Autodesk Fusion 360 part; units mm, degrees
(part 5 of 6)
  arc A300 (17.675, -158.5) -> (14.5, -161.675) centre (17.675, -161.675) ccw
  line L301 (17.675, -158.5) -> (30.325, -158.5)
  arc A301 (33.5, -161.675) -> (30.325, -158.5) centre (30.325, -161.675) ccw
  line L302 (33.5, -161.675) -> (33.5, -174.325)
  arc A302 (30.325, -177.5) -> (33.5, -174.325) centre (30.325, -174.325) ccw
  line L303 (30.325, -177.5) -> (17.675, -177.5)
  arc A303 (14.5, -174.325) -> (17.675, -177.5) centre (17.675, -174.325) ccw
  line L304 (-105.5, -126.325) -> (-105.5, -113.675)
  arc A304 (-102.325, -110.5) -> (-105.5, -113.675) centre (-102.325, -113.675) ccw
  line L305 (-102.325, -110.5) -> (-89.675, -110.5)
  arc A305 (-86.5, -113.675) -> (-89.675, -110.5) centre (-89.675, -113.675) ccw
  line L306 (-86.5, -113.675) -> (-86.5, -126.325)
  arc A306 (-89.675, -129.5) -> (-86.5, -126.325) centre (-89.675, -126.325) ccw
  line L307 (-89.675, -129.5) -> (-102.325, -129.5)
  arc A307 (-105.5, -126.325) -> (-102.325, -129.5) centre (-102.325, -126.325) ccw
  line L308 (-81.5, -6.325) -> (-81.5, 6.325)
  arc A308 (-78.325, 9.5) -> (-81.5, 6.325) centre (-78.325, 6.325) ccw
  line L309 (-78.325, 9.5) -> (-65.675, 9.5)
  arc A309 (-62.5, 6.325) -> (-65.675, 9.5) centre (-65.675, 6.325) ccw
  line L310 (-62.5, 6.325) -> (-62.5, -6.325)
  arc A310 (-65.675, -9.5) -> (-62.5, -6.325) centre (-65.675, -6.325) ccw
  line L311 (-65.675, -9.5) -> (-78.325, -9.5)
  arc A311 (-81.5, -6.325) -> (-78.325, -9.5) centre (-78.325, -6.325) ccw
  line L312 (-33.5, -102.325) -> (-33.5, -89.675)
  arc A312 (-30.325, -86.5) -> (-33.5, -89.675) centre (-30.325, -89.675) ccw
  line L313 (-30.325, -86.5) -> (-17.675, -86.5)
  arc A313 (-14.5, -89.675) -> (-17.675, -86.5) centre (-17.675, -89.675) ccw
  line L314 (-14.5, -89.675) -> (-14.5, -102.325)
  arc A314 (-17.675, -105.5) -> (-14.5, -102.325) centre (-17.675, -102.325) ccw
  line L315 (-17.675, -105.5) -> (-30.325, -105.5)
  arc A315 (-33.5, -102.325) -> (-30.325, -105.5) centre (-30.325, -102.325) ccw
  line L316 (-81.5, -126.325) -> (-81.5, -113.675)
  arc A316 (-78.325, -110.5) -> (-81.5, -113.675) centre (-78.325, -113.675) ccw
  line L317 (-78.325, -110.5) -> (-65.675, -110.5)
  arc A317 (-62.5, -113.675) -> (-65.675, -110.5) centre (-65.675, -113.675) ccw
  line L318 (-62.5, -113.675) -> (-62.5, -126.325)
  arc A318 (-65.675, -129.5) -> (-62.5, -126.325) centre (-65.675, -126.325) ccw
  line L319 (-65.675, -129.5) -> (-78.325, -129.5)
  arc A319 (-81.5, -126.325) -> (-78.325, -129.5) centre (-78.325, -126.325) ccw
  line L320 (38.5, 161.675) -> (38.5, 174.325)
  arc A320 (41.675, 177.5) -> (38.5, 174.325) centre (41.675, 174.325) ccw
  line L321 (41.675, 177.5) -> (54.325, 177.5)
  arc A321 (57.5, 174.325) -> (54.325, 177.5) centre (54.325, 174.325) ccw
  line L322 (57.5, 174.325) -> (57.5, 161.675)
  arc A322 (54.325, 158.5) -> (57.5, 161.675) centre (54.325, 161.675) ccw
  line L323 (54.325, 158.5) -> (41.675, 158.5)
  arc A323 (38.5, 161.675) -> (41.675, 158.5) centre (41.675, 161.675) ccw
  line L324 (38.5, 137.675) -> (38.5, 150.325)
  arc A324 (41.675, 153.5) -> (38.5, 150.325) centre (41.675, 150.325) ccw
  line L325 (41.675, 153.5) -> (54.325, 153.5)
  arc A325 (57.5, 150.325) -> (54.325, 153.5) centre (54.325, 150.325) ccw
  line L326 (57.5, 150.325) -> (57.5, 137.675)
  arc A326 (54.325, 134.5) -> (57.5, 137.675) centre (54.325, 137.675) ccw
  line L327 (54.325, 134.5) -> (41.675, 134.5)
  arc A327 (38.5, 137.675) -> (41.675, 134.5) centre (41.675, 137.675) ccw
  line L328 (38.5, 113.675) -> (38.5, 126.325)
  arc A328 (41.675, 129.5) -> (38.5, 126.325) centre (41.675, 126.325) ccw
  line L329 (41.675, 129.5) -> (54.325, 129.5)
  arc A329 (57.5, 126.325) -> (54.325, 129.5) centre (54.325, 126.325) ccw
  line L330 (57.5, 126.325) -> (57.5, 113.675)
  arc A330 (54.325, 110.5) -> (57.5, 113.675) centre (54.325, 113.675) ccw
  line L331 (54.325, 110.5) -> (41.675, 110.5)
  arc A331 (38.5, 113.675) -> (41.675, 110.5) centre (41.675, 113.675) ccw
  line L332 (38.5, 89.675) -> (38.5, 102.325)
  arc A332 (41.675, 105.5) -> (38.5, 102.325) centre (41.675, 102.325) ccw
  line L333 (41.675, 105.5) -> (54.325, 105.5)
  arc A333 (57.5, 102.325) -> (54.325, 105.5) centre (54.325, 102.325) ccw
  line L334 (57.5, 102.325) -> (57.5, 89.675)
  arc A334 (54.325, 86.5) -> (57.5, 89.675) centre (54.325, 89.675) ccw
  line L335 (54.325, 86.5) -> (41.675, 86.5)
  arc A335 (38.5, 89.675) -> (41.675, 86.5) centre (41.675, 89.675) ccw
  line L336 (134.5, 161.675) -> (134.5, 174.325)
  arc A336 (137.675, 177.5) -> (134.5, 174.325) centre (137.675, 174.325) ccw
  line L337 (137.675, 177.5) -> (150.325, 177.5)
  arc A337 (153.5, 174.325) -> (150.325, 177.5) centre (150.325, 174.325) ccw
  line L338 (153.5, 174.325) -> (153.5, 161.675)
  arc A338 (150.325, 158.5) -> (153.5, 161.675) centre (150.325, 161.675) ccw
  line L339 (150.325, 158.5) -> (137.675, 158.5)
  arc A339 (134.5, 161.675) -> (137.675, 158.5) centre (137.675, 161.675) ccw
  line L340 (62.5, 41.675) -> (62.5, 54.325)
  arc A340 (65.675, 57.5) -> (62.5, 54.325) centre (65.675, 54.325) ccw
  line L341 (65.675, 57.5) -> (78.325, 57.5)
  arc A341 (81.5, 54.325) -> (78.325, 57.5) centre (78.325, 54.325) ccw
  line L342 (81.5, 54.325) -> (81.5, 41.675)
  arc A342 (78.325, 38.5) -> (81.5, 41.675) centre (78.325, 41.675) ccw
  line L343 (78.325, 38.5) -> (65.675, 38.5)
  arc A343 (62.5, 41.675) -> (65.675, 38.5) centre (65.675, 41.675) ccw
  line L344 (62.5, 17.675) -> (62.5, 30.325)
  arc A344 (65.675, 33.5) -> (62.5, 30.325) centre (65.675, 30.325) ccw
  line L345 (65.675, 33.5) -> (78.325, 33.5)
  arc A345 (81.5, 30.325) -> (78.325, 33.5) centre (78.325, 30.325) ccw
  line L346 (81.5, 30.325) -> (81.5, 17.675)
  arc A346 (78.325, 14.5) -> (81.5, 17.675) centre (78.325, 17.675) ccw
  line L347 (78.325, 14.5) -> (65.675, 14.5)
  arc A347 (62.5, 17.675) -> (65.675, 14.5) centre (65.675, 17.675) ccw
  line L348 (62.5, -6.325) -> (62.5, 6.325)
  arc A348 (65.675, 9.5) -> (62.5, 6.325) centre (65.675, 6.325) ccw
  line L349 (65.675, 9.5) -> (78.325, 9.5)
  arc A349 (81.5, 6.325) -> (78.325, 9.5) centre (78.325, 6.325) ccw
  line L350 (81.5, 6.325) -> (81.5, -6.325)
  arc A350 (78.325, -9.5) -> (81.5, -6.325) centre (78.325, -6.325) ccw
  line L351 (78.325, -9.5) -> (65.675, -9.5)
  arc A351 (62.5, -6.325) -> (65.675, -9.5) centre (65.675, -6.325) ccw
  line L352 (158.5, 161.675) -> (158.5, 174.325)
  arc A352 (161.675, 177.5) -> (158.5, 174.325) centre (161.675, 174.325) ccw
  line L353 (161.675, 177.5) -> (174.325, 177.5)
  arc A353 (177.5, 174.325) -> (174.325, 177.5) centre (174.325, 174.325) ccw
  line L354 (177.5, 174.325) -> (177.5, 161.675)
  arc A354 (174.325, 158.5) -> (177.5, 161.675) centre (174.325, 161.675) ccw
  line L355 (174.325, 158.5) -> (161.675, 158.5)
  arc A355 (158.5, 161.675) -> (161.675, 158.5) centre (161.675, 161.675) ccw
  line L356 (134.5, 137.675) -> (134.5, 150.325)
  arc A356 (137.675, 153.5) -> (134.5, 150.325) centre (137.675, 150.325) ccw
  line L357 (137.675, 153.5) -> (150.325, 153.5)
  arc A357 (153.5, 150.325) -> (150.325, 153.5) centre (150.325, 150.325) ccw
  line L358 (153.5, 150.325) -> (153.5, 137.675)
  arc A358 (150.325, 134.5) -> (153.5, 137.675) centre (150.325, 137.675) ccw
  line L359 (150.325, 134.5) -> (137.675, 134.5)
  arc A359 (134.5, 137.675) -> (137.675, 134.5) centre (137.675, 137.675) ccw
  line L360 (134.5, 113.675) -> (134.5, 126.325)
  arc A360 (137.675, 129.5) -> (134.5, 126.325) centre (137.675, 126.325) ccw
  line L361 (137.675, 129.5) -> (150.325, 129.5)
  arc A361 (153.5, 126.325) -> (150.325, 129.5) centre (150.325, 126.325) ccw
  line L362 (153.5, 126.325) -> (153.5, 113.675)
  arc A362 (150.325, 110.5) -> (153.5, 113.675) centre (150.325, 113.675) ccw
  line L363 (150.325, 110.5) -> (137.675, 110.5)
  arc A363 (134.5, 113.675) -> (137.675, 110.5) centre (137.675, 113.675) ccw
  line L364 (134.5, 89.675) -> (134.5, 102.325)
  arc A364 (137.675, 105.5) -> (134.5, 102.325) centre (137.675, 102.325) ccw
  line L365 (137.675, 105.5) -> (150.325, 105.5)
  arc A365 (153.5, 102.325) -> (150.325, 105.5) centre (150.325, 102.325) ccw
  line L366 (153.5, 102.325) -> (153.5, 89.675)
  arc A366 (150.325, 86.5) -> (153.5, 89.675) centre (150.325, 89.675) ccw
  line L367 (150.325, 86.5) -> (137.675, 86.5)
  arc A367 (134.5, 89.675) -> (137.675, 86.5) centre (137.675, 89.675) ccw
  line L368 (134.5, 65.675) -> (134.5, 78.325)
  arc A368 (137.675, 81.5) -> (134.5, 78.325) centre (137.675, 78.325) ccw
  line L369 (137.675, 81.5) -> (150.325, 81.5)
  arc A369 (153.5, 78.325) -> (150.325, 81.5) centre (150.325, 78.325) ccw
  line L370 (153.5, 78.325) -> (153.5, 65.675)
  arc A370 (150.325, 62.5) -> (153.5, 65.675) centre (150.325, 65.675) ccw
  line L371 (150.325, 62.5) -> (137.675, 62.5)
  arc A371 (134.5, 65.675) -> (137.675, 62.5) centre (137.675, 65.675) ccw
  line L372 (134.5, 41.675) -> (134.5, 54.325)
  arc A372 (137.675, 57.5) -> (134.5, 54.325) centre (137.675, 54.325) ccw
  line L373 (137.675, 57.5) -> (150.325, 57.5)
  arc A373 (153.5, 54.325) -> (150.325, 57.5) centre (150.325, 54.325) ccw
  line L374 (153.5, 54.325) -> (153.5, 41.675)
  arc A374 (150.325, 38.5) -> (153.5, 41.675) centre (150.325, 41.675) ccw
  line L375 (150.325, 38.5) -> (137.675, 38.5)
  arc A375 (134.5, 41.675) -> (137.675, 38.5) centre (137.675, 41.675) ccw
  line L376 (134.5, 17.675) -> (134.5, 30.325)
  arc A376 (137.675, 33.5) -> (134.5, 30.325) centre (137.675, 30.325) ccw
  line L377 (137.675, 33.5) -> (150.325, 33.5)
  arc A377 (153.5, 30.325) -> (150.325, 33.5) centre (150.325, 30.325) ccw
  line L378 (153.5, 30.325) -> (153.5, 17.675)
  arc A378 (150.325, 14.5) -> (153.5, 17.675) centre (150.325, 17.675) ccw
  line L379 (150.325, 14.5) -> (137.675, 14.5)
  arc A379 (134.5, 17.675) -> (137.675, 14.5) centre (137.675, 17.675) ccw
  line L380 (134.5, -6.325) -> (134.5, 6.325)
  arc A380 (137.675, 9.5) -> (134.5, 6.325) centre (137.675, 6.325) ccw
  line L381 (137.675, 9.5) -> (150.325, 9.5)
  arc A381 (153.5, 6.325) -> (150.325, 9.5) centre (150.325, 6.325) ccw
  line L382 (153.5, 6.325) -> (153.5, -6.325)
  arc A382 (150.325, -9.5) -> (153.5, -6.325) centre (150.325, -6.325) ccw
  line L383 (150.325, -9.5) -> (137.675, -9.5)
  arc A383 (134.5, -6.325) -> (137.675, -9.5) centre (137.675, -6.325) ccw
  line L384 (38.5, -30.325) -> (38.5, -17.675)
  arc A384 (41.675, -14.5) -> (38.5, -17.675) centre (41.675, -17.675) ccw
  line L385 (41.675, -14.5) -> (54.325, -14.5)
  arc A385 (57.5, -17.675) -> (54.325, -14.5) centre (54.325, -17.675) ccw
  line L386 (57.5, -17.675) -> (57.5, -30.325)
  arc A386 (54.325, -33.5) -> (57.5, -30.325) centre (54.325, -30.325) ccw
  line L387 (54.325, -33.5) -> (41.675, -33.5)
  arc A387 (38.5, -30.325) -> (41.675, -33.5) centre (41.675, -30.325) ccw
  line L388 (38.5, -54.325) -> (38.5, -41.675)
  arc A388 (41.675, -38.5) -> (38.5, -41.675) centre (41.675, -41.675) ccw
  line L389 (41.675, -38.5) -> (54.325, -38.5)
  arc A389 (57.5, -41.675) -> (54.325, -38.5) centre (54.325, -41.675) ccw
  line L390 (57.5, -41.675) -> (57.5, -54.325)
  arc A390 (54.325, -57.5) -> (57.5, -54.325) centre (54.325, -54.325) ccw
  line L391 (54.325, -57.5) -> (41.675, -57.5)
  arc A391 (38.5, -54.325) -> (41.675, -57.5) centre (41.675, -54.325) ccw
  line L392 (-9.5, -102.325) -> (-9.5, -89.675)
  arc A392 (-6.325, -86.5) -> (-9.5, -89.675) centre (-6.325, -89.675) ccw
  line L393 (-6.325, -86.5) -> (6.325, -86.5)
  arc A393 (9.5, -89.675) -> (6.325, -86.5) centre (6.325, -89.675) ccw
  line L394 (9.5, -89.675) -> (9.5, -102.325)
  arc A394 (6.325, -105.5) -> (9.5, -102.325) centre (6.325, -102.325) ccw
  line L395 (6.325, -105.5) -> (-6.325, -105.5)
  arc A395 (-9.5, -102.325) -> (-6.325, -105.5) centre (-6.325, -102.325) ccw
  line L396 (134.5, -78.325) -> (134.5, -65.675)
  arc A396 (137.675, -62.5) -> (134.5, -65.675) centre (137.675, -65.675) ccw
  line L397 (137.675, -62.5) -> (150.325, -62.5)
  arc A397 (153.5, -65.675) -> (150.325, -62.5) centre (150.325, -65.675) ccw
  line L398 (153.5, -65.675) -> (153.5, -78.325)
  arc A398 (150.325, -81.5) -> (153.5, -78.325) centre (150.325, -78.325) ccw
  line L399 (150.325, -81.5) -> (137.675, -81.5)
  arc A399 (134.5, -78.325) -> (137.675, -81.5) centre (137.675, -78.325) ccw
  line L400 (-33.5, 17.675) -> (-33.5, 30.325)
  arc A400 (-30.325, 33.5) -> (-33.5, 30.325) centre (-30.325, 30.325) ccw
  line L401 (-30.325, 33.5) -> (-17.675, 33.5)
  arc A401 (-14.5, 30.325) -> (-17.675, 33.5) centre (-17.675, 30.325) ccw
  line L402 (-14.5, 30.325) -> (-14.5, 17.675)
  arc A402 (-17.675, 14.5) -> (-14.5, 17.675) centre (-17.675, 17.675) ccw
  line L403 (-17.675, 14.5) -> (-30.325, 14.5)
  arc A403 (-33.5, 17.675) -> (-30.325, 14.5) centre (-30.325, 17.675) ccw
  line L404 (62.5, -78.325) -> (62.5, -65.675)
  arc A404 (65.675, -62.5) -> (62.5, -65.675) centre (65.675, -65.675) ccw
  line L405 (65.675, -62.5) -> (78.325, -62.5)
  arc A405 (81.5, -65.675) -> (78.325, -62.5) centre (78.325, -65.675) ccw
  line L406 (81.5, -65.675) -> (81.5, -78.325)
  arc A406 (78.325, -81.5) -> (81.5, -78.325) centre (78.325, -78.325) ccw
  line L407 (78.325, -81.5) -> (65.675, -81.5)
  arc A407 (62.5, -78.325) -> (65.675, -81.5) centre (65.675, -78.325) ccw
  line L408 (-153.5, 17.675) -> (-153.5, 30.325)
  arc A408 (-150.325, 33.5) -> (-153.5, 30.325) centre (-150.325, 30.325) ccw
  line L409 (-150.325, 33.5) -> (-137.675, 33.5)
  arc A409 (-134.5, 30.325) -> (-137.675, 33.5) centre (-137.675, 30.325) ccw
  line L410 (-134.5, 30.325) -> (-134.5, 17.675)
  arc A410 (-137.675, 14.5) -> (-134.5, 17.675) centre (-137.675, 17.675) ccw
  line L411 (-137.675, 14.5) -> (-150.325, 14.5)
  arc A411 (-153.5, 17.675) -> (-150.325, 14.5) centre (-150.325, 17.675) ccw
  line L412 (-129.5, -54.325) -> (-129.5, -41.675)
  arc A412 (-126.325, -38.5) -> (-129.5, -41.675) centre (-126.325, -41.675) ccw
  line L413 (-126.325, -38.5) -> (-113.675, -38.5)
  arc A413 (-110.5, -41.675) -> (-113.675, -38.5) centre (-113.675, -41.675) ccw
  line L414 (-110.5, -41.675) -> (-110.5, -54.325)
  arc A414 (-113.675, -57.5) -> (-110.5, -54.325) centre (-113.675, -54.325) ccw
  line L415 (-113.675, -57.5) -> (-126.325, -57.5)
  arc A415 (-129.5, -54.325) -> (-126.325, -57.5) centre (-126.325, -54.325) ccw
  line L416 (-33.5, -30.325) -> (-33.5, -17.675)
  arc A416 (-30.325, -14.5) -> (-33.5, -17.675) centre (-30.325, -17.675) ccw
  line L417 (-30.325, -14.5) -> (-17.675, -14.5)
  arc A417 (-14.5, -17.675) -> (-17.675, -14.5) centre (-17.675, -17.675) ccw
  line L418 (-14.5, -17.675) -> (-14.5, -30.325)
  arc A418 (-17.675, -33.5) -> (-14.5, -30.325) centre (-17.675, -30.325) ccw
  line L419 (-17.675, -33.5) -> (-30.325, -33.5)
  arc A419 (-33.5, -30.325) -> (-30.325, -33.5) centre (-30.325, -30.325) ccw
  line L420 (158.5, -102.325) -> (158.5, -89.675)
  arc A420 (161.675, -86.5) -> (158.5, -89.675) centre (161.675, -89.675) ccw
  line L421 (161.675, -86.5) -> (174.325, -86.5)
  arc A421 (177.5, -89.675) -> (174.325, -86.5) centre (174.325, -89.675) ccw
  line L422 (177.5, -89.675) -> (177.5, -102.325)
  arc A422 (174.325, -105.5) -> (177.5, -102.325) centre (174.325, -102.325) ccw
  line L423 (174.325, -105.5) -> (161.675, -105.5)
  arc A423 (158.5, -102.325) -> (161.675, -105.5) centre (161.675, -102.325) ccw
  line L424 (-9.5, -126.325) -> (-9.5, -113.675)
  arc A424 (-6.325, -110.5) -> (-9.5, -113.675) centre (-6.325, -113.675) ccw
  line L425 (-6.325, -110.5) -> (6.325, -110.5)
  arc A425 (9.5, -113.675) -> (6.325, -110.5) centre (6.325, -113.675) ccw
  line L426 (9.5, -113.675) -> (9.5, -126.325)
  arc A426 (6.325, -129.5) -> (9.5, -126.325) centre (6.325, -126.325) ccw
  line L427 (6.325, -129.5) -> (-6.325, -129.5)
  arc A427 (-9.5, -126.325) -> (-6.325, -129.5) centre (-6.325, -126.325) ccw
  line L428 (134.5, -30.325) -> (134.5, -17.675)
  arc A428 (137.675, -14.5) -> (134.5, -17.675) centre (137.675, -17.675) ccw
  line L429 (137.675, -14.5) -> (150.325, -14.5)
  arc A429 (153.5, -17.675) -> (150.325, -14.5) centre (150.325, -17.675) ccw
  line L430 (153.5, -17.675) -> (153.5, -30.325)
  arc A430 (150.325, -33.5) -> (153.5, -30.325) centre (150.325, -30.325) ccw
  line L431 (150.325, -33.5) -> (137.675, -33.5)
  arc A431 (134.5, -30.325) -> (137.675, -33.5) centre (137.675, -30.325) ccw
  line L432 (-57.5, 17.675) -> (-57.5, 30.325)
  arc A432 (-54.325, 33.5) -> (-57.5, 30.325) centre (-54.325, 30.325) ccw
  line L433 (-54.325, 33.5) -> (-41.675, 33.5)
  arc A433 (-38.5, 30.325) -> (-41.675, 33.5) centre (-41.675, 30.325) ccw
  line L434 (-38.5, 30.325) -> (-38.5, 17.675)
  arc A434 (-41.675, 14.5) -> (-38.5, 17.675) centre (-41.675, 17.675) ccw
  line L435 (-41.675, 14.5) -> (-54.325, 14.5)
  arc A435 (-57.5, 17.675) -> (-54.325, 14.5) centre (-54.325, 17.675) ccw
  line L436 (-57.5, -30.325) -> (-57.5, -17.675)
  arc A436 (-54.325, -14.5) -> (-57.5, -17.675) centre (-54.325, -17.675) ccw
  line L437 (-54.325, -14.5) -> (-41.675, -14.5)
  arc A437 (-38.5, -17.675) -> (-41.675, -14.5) centre (-41.675, -17.675) ccw
  line L438 (-38.5, -17.675) -> (-38.5, -30.325)
  arc A438 (-41.675, -33.5) -> (-38.5, -30.325) centre (-41.675, -30.325) ccw
  line L439 (-41.675, -33.5) -> (-54.325, -33.5)
  arc A439 (-57.5, -30.325) -> (-54.325, -33.5) centre (-54.325, -30.325) ccw
  line L440 (-57.5, -54.325) -> (-57.5, -41.675)
  arc A440 (-54.325, -38.5) -> (-57.5, -41.675) centre (-54.325, -41.675) ccw
  line L441 (-54.325, -38.5) -> (-41.675, -38.5)
  arc A441 (-38.5, -41.675) -> (-41.675, -38.5) centre (-41.675, -41.675) ccw
  line L442 (-38.5, -41.675) -> (-38.5, -54.325)
  arc A442 (-41.675, -57.5) -> (-38.5, -54.325) centre (-41.675, -54.325) ccw
  line L443 (-41.675, -57.5) -> (-54.325, -57.5)
  arc A443 (-57.5, -54.325) -> (-54.325, -57.5) centre (-54.325, -54.325) ccw
  line L444 (-81.5, -54.325) -> (-81.5, -41.675)
  arc A444 (-78.325, -38.5) -> (-81.5, -41.675) centre (-78.325, -41.675) ccw
  line L445 (-78.325, -38.5) -> (-65.675, -38.5)
  arc A445 (-62.5, -41.675) -> (-65.675, -38.5) centre (-65.675, -41.675) ccw
  line L446 (-62.5, -41.675) -> (-62.5, -54.325)
  arc A446 (-65.675, -57.5) -> (-62.5, -54.325) centre (-65.675, -54.325) ccw
  line L447 (-65.675, -57.5) -> (-78.325, -57.5)
  arc A447 (-81.5, -54.325) -> (-78.325, -57.5) centre (-78.325, -54.325) ccw
  line L448 (14.5, -54.325) -> (14.5, -41.675)
  arc A448 (17.675, -38.5) -> (14.5, -41.675) centre (17.675, -41.675) ccw
  line L449 (17.675, -38.5) -> (30.325, -38.5)
  arc A449 (33.5, -41.675) -> (30.325, -38.5) centre (30.325, -41.675) ccw
  line L450 (33.5, -41.675) -> (33.5, -54.325)
  arc A450 (30.325, -57.5) -> (33.5, -54.325) centre (30.325, -54.325) ccw
  line L451 (30.325, -57.5) -> (17.675, -57.5)
  arc A451 (14.5, -54.325) -> (17.675, -57.5) centre (17.675, -54.325) ccw
  line L452 (86.5, -150.325) -> (86.5, -137.675)
  arc A452 (89.675, -134.5) -> (86.5, -137.675) centre (89.675, -137.675) ccw
  line L453 (89.675, -134.5) -> (102.325, -134.5)
  arc A453 (105.5, -137.675) -> (102.325, -134.5) centre (102.325, -137.675) ccw
  line L454 (105.5, -137.675) -> (105.5, -150.325)
  arc A454 (102.325, -153.5) -> (105.5, -150.325) centre (102.325, -150.325) ccw
  line L455 (102.325, -153.5) -> (89.675, -153.5)
  arc A455 (86.5, -150.325) -> (89.675, -153.5) centre (89.675, -150.325) ccw
  line L456 (158.5, -54.325) -> (158.5, -41.675)
  arc A456 (161.675, -38.5) -> (158.5, -41.675) centre (161.675, -41.675) ccw
  line L457 (161.675, -38.5) -> (174.325, -38.5)
  arc A457 (177.5, -41.675) -> (174.325, -38.5) centre (174.325, -41.675) ccw
  line L458 (177.5, -41.675) -> (177.5, -54.325)
  arc A458 (174.325, -57.5) -> (177.5, -54.325) centre (174.325, -54.325) ccw
  line L459 (174.325, -57.5) -> (161.675, -57.5)
  arc A459 (158.5, -54.325) -> (161.675, -57.5) centre (161.675, -54.325) ccw
  line L460 (-129.5, -6.325) -> (-129.5, 6.325)
  arc A460 (-126.325, 9.5) -> (-129.5, 6.325) centre (-126.325, 6.325) ccw
  line L461 (-126.325, 9.5) -> (-113.675, 9.5)
  arc A461 (-110.5, 6.325) -> (-113.675, 9.5) centre (-113.675, 6.325) ccw
  line L462 (-110.5, 6.325) -> (-110.5, -6.325)
  arc A462 (-113.675, -9.5) -> (-110.5, -6.325) centre (-113.675, -6.325) ccw
  line L463 (-113.675, -9.5) -> (-126.325, -9.5)
  arc A463 (-129.5, -6.325) -> (-126.325, -9.5) centre (-126.325, -6.325) ccw
  line L464 (-57.5, -6.325) -> (-57.5, 6.325)
  arc A464 (-54.325, 9.5) -> (-57.5, 6.325) centre (-54.325, 6.325) ccw
  line L465 (-54.325, 9.5) -> (-41.675, 9.5)
  arc A465 (-38.5, 6.325) -> (-41.675, 9.5) centre (-41.675, 6.325) ccw
  line L466 (-38.5, 6.325) -> (-38.5, -6.325)
  arc A466 (-41.675, -9.5) -> (-38.5, -6.325) centre (-41.675, -6.325) ccw
  line L467 (-41.675, -9.5) -> (-54.325, -9.5)
  arc A467 (-57.5, -6.325) -> (-54.325, -9.5) centre (-54.325, -6.325) ccw
  line L468 (14.5, -126.325) -> (14.5, -113.675)
  arc A468 (17.675, -110.5) -> (14.5, -113.675) centre (17.675, -113.675) ccw
  line L469 (17.675, -110.5) -> (30.325, -110.5)
  arc A469 (33.5, -113.675) -> (30.325, -110.5) centre (30.325, -113.675) ccw
  line L470 (33.5, -113.675) -> (33.5, -126.325)
  arc A470 (30.325, -129.5) -> (33.5, -126.325) centre (30.325, -126.325) ccw
  line L471 (30.325, -129.5) -> (17.675, -129.5)
  arc A471 (14.5, -126.325) -> (17.675, -129.5) centre (17.675, -126.325) ccw
  line L472 (-9.5, -150.325) -> (-9.5, -137.675)
  arc A472 (-6.325, -134.5) -> (-9.5, -137.675) centre (-6.325, -137.675) ccw
  line L473 (-6.325, -134.5) -> (6.325, -134.5)
  arc A473 (9.5, -137.675) -> (6.325, -134.5) centre (6.325, -137.675) ccw
  line L474 (9.5, -137.675) -> (9.5, -150.325)
  arc A474 (6.325, -153.5) -> (9.5, -150.325) centre (6.325, -150.325) ccw
  line L475 (6.325, -153.5) -> (-6.325, -153.5)
  arc A475 (-9.5, -150.325) -> (-6.325, -153.5) centre (-6.325, -150.325) ccw
  line L476 (110.5, -30.325) -> (110.5, -17.675)
  arc A476 (113.675, -14.5) -> (110.5, -17.675) centre (113.675, -17.675) ccw
  line L477 (113.675, -14.5) -> (126.325, -14.5)
  arc A477 (129.5, -17.675) -> (126.325, -14.5) centre (126.325, -17.675) ccw
  line L478 (129.5, -17.675) -> (129.5, -30.325)
  arc A478 (126.325, -33.5) -> (129.5, -30.325) centre (126.325, -30.325) ccw
  line L479 (126.325, -33.5) -> (113.675, -33.5)
  arc A479 (110.5, -30.325) -> (113.675, -33.5) centre (113.675, -30.325) ccw
  line L480 (-129.5, 17.675) -> (-129.5, 30.325)
  arc A480 (-126.325, 33.5) -> (-129.5, 30.325) centre (-126.325, 30.325) ccw
  line L481 (-126.325, 33.5) -> (-113.675, 33.5)
  arc A481 (-110.5, 30.325) -> (-113.675, 33.5) centre (-113.675, 30.325) ccw
  line L482 (-110.5, 30.325) -> (-110.5, 17.675)
  arc A482 (-113.675, 14.5) -> (-110.5, 17.675) centre (-113.675, 17.675) ccw
  line L483 (-113.675, 14.5) -> (-126.325, 14.5)
  arc A483 (-129.5, 17.675) -> (-126.325, 14.5) centre (-126.325, 17.675) ccw
  line L484 (-33.5, -150.325) -> (-33.5, -137.675)
  arc A484 (-30.325, -134.5) -> (-33.5, -137.675) centre (-30.325, -137.675) ccw
  line L485 (-30.325, -134.5) -> (-17.675, -134.5)
  arc A485 (-14.5, -137.675) -> (-17.675, -134.5) centre (-17.675, -137.675) ccw
  line L486 (-14.5, -137.675) -> (-14.5, -150.325)
  arc A486 (-17.675, -153.5) -> (-14.5, -150.325) centre (-17.675, -150.325) ccw
  line L487 (-17.675, -153.5) -> (-30.325, -153.5)
  arc A487 (-33.5, -150.325) -> (-30.325, -153.5) centre (-30.325, -150.325) ccw
  line L488 (-57.5, -150.325) -> (-57.5, -137.675)
  arc A488 (-54.325, -134.5) -> (-57.5, -137.675) centre (-54.325, -137.675) ccw
  line L489 (-54.325, -134.5) -> (-41.675, -134.5)
  arc A489 (-38.5, -137.675) -> (-41.675, -134.5) centre (-41.675, -137.675) ccw
  line L490 (-38.5, -137.675) -> (-38.5, -150.325)
  arc A490 (-41.675, -153.5) -> (-38.5, -150.325) centre (-41.675, -150.325) ccw
  line L491 (-41.675, -153.5) -> (-54.325, -153.5)
  arc A491 (-57.5, -150.325) -> (-54.325, -153.5) centre (-54.325, -150.325) ccw
  line L492 (134.5, -150.325) -> (134.5, -137.675)
  arc A492 (137.675, -134.5) -> (134.5, -137.675) centre (137.675, -137.675) ccw
  line L493 (137.675, -134.5) -> (150.325, -134.5)
  arc A493 (153.5, -137.675) -> (150.325, -134.5) centre (150.325, -137.675) ccw
  line L494 (153.5, -137.675) -> (153.5, -150.325)
  arc A494 (150.325, -153.5) -> (153.5, -150.325) centre (150.325, -150.325) ccw
  line L495 (150.325, -153.5) -> (137.675, -153.5)
  arc A495 (134.5, -150.325) -> (137.675, -153.5) centre (137.675, -150.325) ccw
  line L496 (158.5, -174.325) -> (158.5, -161.675)
  arc A496 (161.675, -158.5) -> (158.5, -161.675) centre (161.675, -161.675) ccw
  line L497 (161.675, -158.5) -> (174.325, -158.5)
  arc A497 (177.5, -161.675) -> (174.325, -158.5) centre (174.325, -161.675) ccw
  line L498 (177.5, -161.675) -> (177.5, -174.325)
  arc A498 (174.325, -177.5) -> (177.5, -174.325) centre (174.325, -174.325) ccw
  line L499 (174.325, -177.5) -> (161.675, -177.5)
  arc A499 (158.5, -174.325) -> (161.675, -177.5) centre (161.675, -174.325) ccw
  line L500 (86.5, -78.325) -> (86.5, -65.675)
  arc A500 (89.675, -62.5) -> (86.5, -65.675) centre (89.675, -65.675) ccw
  line L501 (89.675, -62.5) -> (102.325, -62.5)
  arc A501 (105.5, -65.675) -> (102.325, -62.5) centre (102.325, -65.675) ccw
  line L502 (105.5, -65.675) -> (105.5, -78.325)
  arc A502 (102.325, -81.5) -> (105.5, -78.325) centre (102.325, -78.325) ccw
  line L503 (102.325, -81.5) -> (89.675, -81.5)
  arc A503 (86.5, -78.325) -> (89.675, -81.5) centre (89.675, -78.325) ccw
  line L504 (62.5, -174.325) -> (62.5, -161.675)
  arc A504 (65.675, -158.5) -> (62.5, -161.675) centre (65.675, -161.675) ccw
  line L505 (65.675, -158.5) -> (78.325, -158.5)
  arc A505 (81.5, -161.675) -> (78.325, -158.5) centre (78.325, -161.675) ccw
  line L506 (81.5, -161.675) -> (81.5, -174.325)
  arc A506 (78.325, -177.5) -> (81.5, -174.325) centre (78.325, -174.325) ccw
  line L507 (78.325, -177.5) -> (65.675, -177.5)
  arc A507 (62.5, -174.325) -> (65.675, -177.5) centre (65.675, -174.325) ccw
  line L508 (38.5, -102.325) -> (38.5, -89.675)
  arc A508 (41.675, -86.5) -> (38.5, -89.675) centre (41.675, -89.675) ccw
  line L509 (41.675, -86.5) -> (54.325, -86.5)
  arc A509 (57.5, -89.675) -> (54.325, -86.5) centre (54.325, -89.675) ccw
  line L510 (57.5, -89.675) -> (57.5, -102.325)
  arc A510 (54.325, -105.5) -> (57.5, -102.325) centre (54.325, -102.325) ccw
  line L511 (54.325, -105.5) -> (41.675, -105.5)
  arc A511 (38.5, -102.325) -> (41.675, -105.5) centre (41.675, -102.325) ccw
  line L512 (-9.5, -30.325) -> (-9.5, -17.675)
  arc A512 (-6.325, -14.5) -> (-9.5, -17.675) centre (-6.325, -17.675) ccw
  line L513 (-6.325, -14.5) -> (6.325, -14.5)
  arc A513 (9.5, -17.675) -> (6.325, -14.5) centre (6.325, -17.675) ccw
  line L514 (9.5, -17.675) -> (9.5, -30.325)
  arc A514 (6.325, -33.5) -> (9.5, -30.325) centre (6.325, -30.325) ccw
  line L515 (6.325, -33.5) -> (-6.325, -33.5)
  arc A515 (-9.5, -30.325) -> (-6.325, -33.5) centre (-6.325, -30.325) ccw
  line L516 (86.5, -6.325) -> (86.5, 6.325)
  arc A516 (89.675, 9.5) -> (86.5, 6.325) centre (89.675, 6.325) ccw
  line L517 (89.675, 9.5) -> (102.325, 9.5)
  arc A517 (105.5, 6.325) -> (102.325, 9.5) centre (102.325, 6.325) ccw
  line L518 (105.5, 6.325) -> (105.5, -6.325)
  arc A518 (102.325, -9.5) -> (105.5, -6.325) centre (102.325, -6.325) ccw
  line L519 (102.325, -9.5) -> (89.675, -9.5)
  arc A519 (86.5, -6.325) -> (89.675, -9.5) centre (89.675, -6.325) ccw
  line L520 (86.5, 17.675) -> (86.5, 30.325)
  arc A520 (89.675, 33.5) -> (86.5, 30.325) centre (89.675, 30.325) ccw
  line L521 (89.675, 33.5) -> (102.325, 33.5)
  arc A521 (105.5, 30.325) -> (102.325, 33.5) centre (102.325, 30.325) ccw
  line L522 (105.5, 30.325) -> (105.5, 17.675)
  arc A522 (102.325, 14.5) -> (105.5, 17.675) centre (102.325, 17.675) ccw
  line L523 (102.325, 14.5) -> (89.675, 14.5)
  arc A523 (86.5, 17.675) -> (89.675, 14.5) centre (89.675, 17.675) ccw
  line L524 (86.5, 41.675) -> (86.5, 54.325)
  arc A524 (89.675, 57.5) -> (86.5, 54.325) centre (89.675, 54.325) ccw
  line L525 (89.675, 57.5) -> (102.325, 57.5)
  arc A525 (105.5, 54.325) -> (102.325, 57.5) centre (102.325, 54.325) ccw
  line L526 (105.5, 54.325) -> (105.5, 41.675)
  arc A526 (102.325, 38.5) -> (105.5, 41.675) centre (102.325, 41.675) ccw
  line L527 (102.325, 38.5) -> (89.675, 38.5)
  arc A527 (86.5, 41.675) -> (89.675, 38.5) centre (89.675, 41.675) ccw
  line L528 (86.5, 65.675) -> (86.5, 78.325)
  arc A528 (89.675, 81.5) -> (86.5, 78.325) centre (89.675, 78.325) ccw
  line L529 (89.675, 81.5) -> (102.325, 81.5)
  arc A529 (105.5, 78.325) -> (102.325, 81.5) centre (102.325, 78.325) ccw
  line L530 (105.5, 78.325) -> (105.5, 65.675)
  arc A530 (102.325, 62.5) -> (105.5, 65.675) centre (102.325, 65.675) ccw
  line L531 (102.325, 62.5) -> (89.675, 62.5)
  arc A531 (86.5, 65.675) -> (89.675, 62.5) centre (89.675, 65.675) ccw
  line L532 (86.5, 89.675) -> (86.5, 102.325)
  arc A532 (89.675, 105.5) -> (86.5, 102.325) centre (89.675, 102.325) ccw
  line L533 (89.675, 105.5) -> (102.325, 105.5)
  arc A533 (105.5, 102.325) -> (102.325, 105.5) centre (102.325, 102.325) ccw
  line L534 (105.5, 102.325) -> (105.5, 89.675)
  arc A534 (102.325, 86.5) -> (105.5, 89.675) centre (102.325, 89.675) ccw
  line L535 (102.325, 86.5) -> (89.675, 86.5)
  arc A535 (86.5, 89.675) -> (89.675, 86.5) centre (89.675, 89.675) ccw
  line L536 (86.5, 113.675) -> (86.5, 126.325)
  arc A536 (89.675, 129.5) -> (86.5, 126.325) centre (89.675, 126.325) ccw
  line L537 (89.675, 129.5) -> (102.325, 129.5)
  arc A537 (105.5, 126.325) -> (102.325, 129.5) centre (102.325, 126.325) ccw
  line L538 (105.5, 126.325) -> (105.5, 113.675)
  arc A538 (102.325, 110.5) -> (105.5, 113.675) centre (102.325, 113.675) ccw
  line L539 (102.325, 110.5) -> (89.675, 110.5)
  arc A539 (86.5, 113.675) -> (89.675, 110.5) centre (89.675, 113.675) ccw
  line L540 (86.5, 137.675) -> (86.5, 150.325)
  arc A540 (89.675, 153.5) -> (86.5, 150.325) centre (89.675, 150.325) ccw
  line L541 (89.675, 153.5) -> (102.325, 153.5)
  arc A541 (105.5, 150.325) -> (102.325, 153.5) centre (102.325, 150.325) ccw
  line L542 (105.5, 150.325) -> (105.5, 137.675)
  arc A542 (102.325, 134.5) -> (105.5, 137.675) centre (102.325, 137.675) ccw
  line L543 (102.325, 134.5) -> (89.675, 134.5)
  arc A543 (86.5, 137.675) -> (89.675, 134.5) centre (89.675, 137.675) ccw
  line L544 (86.5, 161.675) -> (86.5, 174.325)
  arc A544 (89.675, 177.5) -> (86.5, 174.325) centre (89.675, 174.325) ccw
  line L545 (89.675, 177.5) -> (102.325, 177.5)
  arc A545 (105.5, 174.325) -> (102.325, 177.5) centre (102.325, 174.325) ccw
  line L546 (105.5, 174.325) -> (105.5, 161.675)
  arc A546 (102.325, 158.5) -> (105.5, 161.675) centre (102.325, 161.675) ccw
  line L547 (102.325, 158.5) -> (89.675, 158.5)
  arc A547 (86.5, 161.675) -> (89.675, 158.5) centre (89.675, 161.675) ccw
  line L548 (14.5, -6.325) -> (14.5, 6.325)
  arc A548 (17.675, 9.5) -> (14.5, 6.325) centre (17.675, 6.325) ccw
  line L549 (17.675, 9.5) -> (30.325, 9.5)
  arc A549 (33.5, 6.325) -> (30.325, 9.5) centre (30.325, 6.325) ccw
  line L550 (33.5, 6.325) -> (33.5, -6.325)
  arc A550 (30.325, -9.5) -> (33.5, -6.325) centre (30.325, -6.325) ccw
  line L551 (30.325, -9.5) -> (17.675, -9.5)
  arc A551 (14.5, -6.325) -> (17.675, -9.5) centre (17.675, -6.325) ccw
  line L552 (14.5, 17.675) -> (14.5, 30.325)
  arc A552 (17.675, 33.5) -> (14.5, 30.325) centre (17.675, 30.325) ccw
  line L553 (17.675, 33.5) -> (30.325, 33.5)
  arc A553 (33.5, 30.325) -> (30.325, 33.5) centre (30.325, 30.325) ccw
  line L554 (33.5, 30.325) -> (33.5, 17.675)
  arc A554 (30.325, 14.5) -> (33.5, 17.675) centre (30.325, 17.675) ccw
  line L555 (30.325, 14.5) -> (17.675, 14.5)
  arc A555 (14.5, 17.675) -> (17.675, 14.5) centre (17.675, 17.675) ccw
  line L556 (14.5, 41.675) -> (14.5, 54.325)
  arc A556 (17.675, 57.5) -> (14.5, 54.325) centre (17.675, 54.325) ccw
  line L557 (17.675, 57.5) -> (30.325, 57.5)
  arc A557 (33.5, 54.325) -> (30.325, 57.5) centre (30.325, 54.325) ccw
  line L558 (33.5, 54.325) -> (33.5, 41.675)
  arc A558 (30.325, 38.5) -> (33.5, 41.675) centre (30.325, 41.675) ccw
  line L559 (30.325, 38.5) -> (17.675, 38.5)
  arc A559 (14.5, 41.675) -> (17.675, 38.5) centre (17.675, 41.675) ccw
  line L560 (14.5, 65.675) -> (14.5, 78.325)
  arc A560 (17.675, 81.5) -> (14.5, 78.325) centre (17.675, 78.325) ccw
  line L561 (17.675, 81.5) -> (30.325, 81.5)
  arc A561 (33.5, 78.325) -> (30.325, 81.5) centre (30.325, 78.325) ccw
  line L562 (33.5, 78.325) -> (33.5, 65.675)
  arc A562 (30.325, 62.5) -> (33.5, 65.675) centre (30.325, 65.675) ccw
  line L563 (30.325, 62.5) -> (17.675, 62.5)
  arc A563 (14.5, 65.675) -> (17.675, 62.5) centre (17.675, 65.675) ccw
  line L564 (-9.5, 89.675) -> (-9.5, 102.325)
  arc A564 (-6.325, 105.5) -> (-9.5, 102.325) centre (-6.325, 102.325) ccw
  line L565 (-6.325, 105.5) -> (6.325, 105.5)
  arc A565 (9.5, 102.325) -> (6.325, 105.5) centre (6.325, 102.325) ccw
  line L566 (9.5, 102.325) -> (9.5, 89.675)
  arc A566 (6.325, 86.5) -> (9.5, 89.675) centre (6.325, 89.675) ccw
  line L567 (6.325, 86.5) -> (-6.325, 86.5)
  arc A567 (-9.5, 89.675) -> (-6.325, 86.5) centre (-6.325, 89.675) ccw
  line L568 (-9.5, 113.675) -> (-9.5, 126.325)
  arc A568 (-6.325, 129.5) -> (-9.5, 126.325) centre (-6.325, 126.325) ccw
  line L569 (-6.325, 129.5) -> (6.325, 129.5)
  arc A569 (9.5, 126.325) -> (6.325, 129.5) centre (6.325, 126.325) ccw
  line L570 (9.5, 126.325) -> (9.5, 113.675)
  arc A570 (6.325, 110.5) -> (9.5, 113.675) centre (6.325, 113.675) ccw
  line L571 (6.325, 110.5) -> (-6.325, 110.5)
  arc A571 (-9.5, 113.675) -> (-6.325, 110.5) centre (-6.325, 113.675) ccw
  line L572 (-9.5, 137.675) -> (-9.5, 150.325)
  arc A572 (-6.325, 153.5) -> (-9.5, 150.325) centre (-6.325, 150.325) ccw
  line L573 (-6.325, 153.5) -> (6.325, 153.5)
  arc A573 (9.5, 150.325) -> (6.325, 153.5) centre (6.325, 150.325) ccw
  line L574 (9.5, 150.325) -> (9.5, 137.675)
  arc A574 (6.325, 134.5) -> (9.5, 137.675) centre (6.325, 137.675) ccw
  line L575 (6.325, 134.5) -> (-6.325, 134.5)
  arc A575 (-9.5, 137.675) -> (-6.325, 134.5) centre (-6.325, 137.675) ccw
  line L576 (14.5, 161.675) -> (14.5, 174.325)
  arc A576 (17.675, 177.5) -> (14.5, 174.325) centre (17.675, 174.325) ccw
  line L577 (17.675, 177.5) -> (30.325, 177.5)
  arc A577 (33.5, 174.325) -> (30.325, 177.5) centre (30.325, 174.325) ccw
  line L578 (33.5, 174.325) -> (33.5, 161.675)
  arc A578 (30.325, 158.5) -> (33.5, 161.675) centre (30.325, 161.675) ccw
  line L579 (30.325, 158.5) -> (17.675, 158.5)
  arc A579 (14.5, 161.675) -> (17.675, 158.5) centre (17.675, 161.675) ccw
  line L580 (-105.5, -78.325) -> (-105.5, -65.675)
  arc A580 (-102.325, -62.5) -> (-105.5, -65.675) centre (-102.325, -65.675) ccw
  line L581 (-102.325, -62.5) -> (-89.675, -62.5)
  arc A581 (-86.5, -65.675) -> (-89.675, -62.5) centre (-89.675, -65.675) ccw
  line L582 (-86.5, -65.675) -> (-86.5, -78.325)
  arc A582 (-89.675, -81.5) -> (-86.5, -78.325) centre (-89.675, -78.325) ccw
  line L583 (-89.675, -81.5) -> (-102.325, -81.5)
  arc A583 (-105.5, -78.325) -> (-102.325, -81.5) centre (-102.325, -78.325) ccw
  line L584 (-105.5, 41.675) -> (-105.5, 54.325)
  arc A584 (-102.325, 57.5) -> (-105.5, 54.325) centre (-102.325, 54.325) ccw
  line L585 (-102.325, 57.5) -> (-89.675, 57.5)
  arc A585 (-86.5, 54.325) -> (-89.675, 57.5) centre (-89.675, 54.325) ccw
  line L586 (-86.5, 54.325) -> (-86.5, 41.675)
  arc A586 (-89.675, 38.5) -> (-86.5, 41.675) centre (-89.675, 41.675) ccw
  line L587 (-89.675, 38.5) -> (-102.325, 38.5)
  arc A587 (-105.5, 41.675) -> (-102.325, 38.5) centre (-102.325, 41.675) ccw
  line L588 (-177.5, -30.325) -> (-177.5, -17.675)
  arc A588 (-174.325, -14.5) -> (-177.5, -17.675) centre (-174.325, -17.675) ccw
  line L589 (-174.325, -14.5) -> (-161.675, -14.5)
  arc A589 (-158.5, -17.675) -> (-161.675, -14.5) centre (-161.675, -17.675) ccw
  line L590 (-158.5, -17.675) -> (-158.5, -30.325)
  arc A590 (-161.675, -33.5) -> (-158.5, -30.325) centre (-161.675, -30.325) ccw
  line L591 (-161.675, -33.5) -> (-174.325, -33.5)
  arc A591 (-177.5, -30.325) -> (-174.325, -33.5) centre (-174.325, -30.325) ccw
  line L592 (-57.5, -174.325) -> (-57.5, -161.675)
  arc A592 (-54.325, -158.5) -> (-57.5, -161.675) centre (-54.325, -161.675) ccw
  line L593 (-54.325, -158.5) -> (-41.675, -158.5)
  arc A593 (-38.5, -161.675) -> (-41.675, -158.5) centre (-41.675, -161.675) ccw
  line L594 (-38.5, -161.675) -> (-38.5, -174.325)
  arc A594 (-41.675, -177.5) -> (-38.5, -174.325) centre (-41.675, -174.325) ccw
  line L595 (-41.675, -177.5) -> (-54.325, -177.5)
  arc A595 (-57.5, -174.325) -> (-54.325, -177.5) centre (-54.325, -174.325) ccw
  line L596 (-105.5, -30.325) -> (-105.5, -17.675)
  arc A596 (-102.325, -14.5) -> (-105.5, -17.675) centre (-102.325, -17.675) ccw
  line L597 (-102.325, -14.5) -> (-89.675, -14.5)
  arc A597 (-86.5, -17.675) -> (-89.675, -14.5) centre (-89.675, -17.675) ccw
  line L598 (-86.5, -17.675) -> (-86.5, -30.325)
  arc A598 (-89.675, -33.5) -> (-86.5, -30.325) centre (-89.675, -30.325) ccw
  line L599 (-89.675, -33.5) -> (-102.325, -33.5)
  arc A599 (-105.5, -30.325) -> (-102.325, -33.5) centre (-102.325, -30.325) ccw
  line L600 (-33.5, -78.325) -> (-33.5, -65.675)
  arc A600 (-30.325, -62.5) -> (-33.5, -65.675) centre (-30.325, -65.675) ccw
  line L601 (-30.325, -62.5) -> (-17.675, -62.5)
  arc A601 (-14.5, -65.675) -> (-17.675, -62.5) centre (-17.675, -65.675) ccw
  line L602 (-14.5, -65.675) -> (-14.5, -78.325)
  arc A602 (-17.675, -81.5) -> (-14.5, -78.325) centre (-17.675, -78.325) ccw
  line L603 (-17.675, -81.5) -> (-30.325, -81.5)
  arc A603 (-33.5, -78.325) -> (-30.325, -81.5) centre (-30.325, -78.325) ccw
  line L604 (-9.5, -54.325) -> (-9.5, -41.675)
  arc A604 (-6.325, -38.5) -> (-9.5, -41.675) centre (-6.325, -41.675) ccw
  line L605 (-6.325, -38.5) -> (6.325, -38.5)
  arc A605 (9.5, -41.675) -> (6.325, -38.5) centre (6.325, -41.675) ccw
  line L606 (9.5, -41.675) -> (9.5, -54.325)
  arc A606 (6.325, -57.5) -> (9.5, -54.325) centre (6.325, -54.325) ccw
  line L607 (6.325, -57.5) -> (-6.325, -57.5)
  arc A607 (-9.5, -54.325) -> (-6.325, -57.5) centre (-6.325, -54.325) ccw
  line L608 (-177.5, -174.325) -> (-177.5, -161.675)
  arc A608 (-174.325, -158.5) -> (-177.5, -161.675) centre (-174.325, -161.675) ccw
  line L609 (-174.325, -158.5) -> (-161.675, -158.5)
  arc A609 (-158.5, -161.675) -> (-161.675, -158.5) centre (-161.675, -161.675) ccw
  line L610 (-158.5, -161.675) -> (-158.5, -174.325)
  arc A610 (-161.675, -177.5) -> (-158.5, -174.325) centre (-161.675, -174.325) ccw
  line L611 (-161.675, -177.5) -> (-174.325, -177.5)
  arc A611 (-177.5, -174.325) -> (-174.325, -177.5) centre (-174.325, -174.325) ccw
  line L612 (-153.5, -150.325) -> (-153.5, -137.675)
  arc A612 (-150.325, -134.5) -> (-153.5, -137.675) centre (-150.325, -137.675) ccw
  line L613 (-150.325, -134.5) -> (-137.675, -134.5)
  arc A613 (-134.5, -137.675) -> (-137.675, -134.5) centre (-137.675, -137.675) ccw
  line L614 (-134.5, -137.675) -> (-134.5, -150.325)
  arc A614 (-137.675, -153.5) -> (-134.5, -150.325) centre (-137.675, -150.325) ccw
  line L615 (-137.675, -153.5) -> (-150.325, -153.5)
  arc A615 (-153.5, -150.325) -> (-150.325, -153.5) centre (-150.325, -150.325) ccw
  line L616 (-129.5, -126.325) -> (-129.5, -113.675)
  arc A616 (-126.325, -110.5) -> (-129.5, -113.675) centre (-126.325, -113.675) ccw
  line L617 (-126.325, -110.5) -> (-113.675, -110.5)
  arc A617 (-110.5, -113.675) -> (-113.675, -110.5) centre (-113.675, -113.675) ccw
  line L618 (-110.5, -113.675) -> (-110.5, -126.325)
  arc A618 (-113.675, -129.5) -> (-110.5, -126.325) centre (-113.675, -126.325) ccw
  line L619 (-113.675, -129.5) -> (-126.325, -129.5)
  arc A619 (-129.5, -126.325) -> (-126.325, -129.5) centre (-126.325, -126.325) ccw
  line L620 (-177.5, -78.325) -> (-177.5, -65.675)
  arc A620 (-174.325, -62.5) -> (-177.5, -65.675) centre (-174.325, -65.675) ccw
  line L621 (-174.325, -62.5) -> (-161.675, -62.5)
  arc A621 (-158.5, -65.675) -> (-161.675, -62.5) centre (-161.675, -65.675) ccw
  line L622 (-158.5, -65.675) -> (-158.5, -78.325)
  arc A622 (-161.675, -81.5) -> (-158.5, -78.325) centre (-161.675, -78.325) ccw
  line L623 (-161.675, -81.5) -> (-174.325, -81.5)
  arc A623 (-177.5, -78.325) -> (-174.325, -81.5) centre (-174.325, -78.325) ccw
  line L624 (-153.5, -54.325) -> (-153.5, -41.675)
  arc A624 (-150.325, -38.5) -> (-153.5, -41.675) centre (-150.325, -41.675) ccw
  line L625 (-150.325, -38.5) -> (-137.675, -38.5)
  arc A625 (-134.5, -41.675) -> (-137.675, -38.5) centre (-137.675, -41.675) ccw
  line L626 (-134.5, -41.675) -> (-134.5, -54.325)
  arc A626 (-137.675, -57.5) -> (-134.5, -54.325) centre (-137.675, -54.325) ccw
  line L627 (-137.675, -57.5) -> (-150.325, -57.5)
  arc A627 (-153.5, -54.325) -> (-150.325, -57.5) centre (-150.325, -54.325) ccw
  line L628 (-129.5, 65.675) -> (-129.5, 78.325)
  arc A628 (-126.325, 81.5) -> (-129.5, 78.325) centre (-126.325, 78.325) ccw
  line L629 (-126.325, 81.5) -> (-113.675, 81.5)
  arc A629 (-110.5, 78.325) -> (-113.675, 81.5) centre (-113.675, 78.325) ccw
  line L630 (-110.5, 78.325) -> (-110.5, 65.675)
  arc A630 (-113.675, 62.5) -> (-110.5, 65.675) centre (-113.675, 65.675) ccw
  line L631 (-113.675, 62.5) -> (-126.325, 62.5)
  arc A631 (-129.5, 65.675) -> (-126.325, 62.5) centre (-126.325, 65.675) ccw
  line L632 (-33.5, 65.675) -> (-33.5, 78.325)
  arc A632 (-30.325, 81.5) -> (-33.5, 78.325) centre (-30.325, 78.325) ccw
  line L633 (-30.325, 81.5) -> (-17.675, 81.5)
  arc A633 (-14.5, 78.325) -> (-17.675, 81.5) centre (-17.675, 78.325) ccw
  line L634 (-14.5, 78.325) -> (-14.5, 65.675)
  arc A634 (-17.675, 62.5) -> (-14.5, 65.675) centre (-17.675, 65.675) ccw
  line L635 (-17.675, 62.5) -> (-30.325, 62.5)
  arc A635 (-33.5, 65.675) -> (-30.325, 62.5) centre (-30.325, 65.675) ccw
  line L636 (-105.5, 89.675) -> (-105.5, 102.325)
  arc A636 (-102.325, 105.5) -> (-105.5, 102.325) centre (-102.325, 102.325) ccw
  line L637 (-102.325, 105.5) -> (-89.675, 105.5)
  arc A637 (-86.5, 102.325) -> (-89.675, 105.5) centre (-89.675, 102.325) ccw
  line L638 (-86.5, 102.325) -> (-86.5, 89.675)
  arc A638 (-89.675, 86.5) -> (-86.5, 89.675) centre (-89.675, 89.675) ccw
  line L639 (-89.675, 86.5) -> (-102.325, 86.5)
  arc A639 (-105.5, 89.675) -> (-102.325, 86.5) centre (-102.325, 89.675) ccw
  line L640 (-177.5, 113.675) -> (-177.5, 126.325)
  arc A640 (-174.325, 129.5) -> (-177.5, 126.325) centre (-174.325, 126.325) ccw
  line L641 (-174.325, 129.5) -> (-161.675, 129.5)
  arc A641 (-158.5, 126.325) -> (-161.675, 129.5) centre (-161.675, 126.325) ccw
  line L642 (-158.5, 126.325) -> (-158.5, 113.675)
  arc A642 (-161.675, 110.5) -> (-158.5, 113.675) centre (-161.675, 113.675) ccw
  line L643 (-161.675, 110.5) -> (-174.325, 110.5)
  arc A643 (-177.5, 113.675) -> (-174.325, 110.5) centre (-174.325, 113.675) ccw
  line L644 (-81.5, 113.675) -> (-81.5, 126.325)
  arc A644 (-78.325, 129.5) -> (-81.5, 126.325) centre (-78.325, 126.325) ccw
  line L645 (-78.325, 129.5) -> (-65.675, 129.5)
  arc A645 (-62.5, 126.325) -> (-65.675, 129.5) centre (-65.675, 126.325) ccw
  line L646 (-62.5, 126.325) -> (-62.5, 113.675)
  arc A646 (-65.675, 110.5) -> (-62.5, 113.675) centre (-65.675, 113.675) ccw
  line L647 (-65.675, 110.5) -> (-78.325, 110.5)
  arc A647 (-81.5, 113.675) -> (-78.325, 110.5) centre (-78.325, 113.675) ccw
  line L648 (-153.5, 137.675) -> (-153.5, 150.325)
  arc A648 (-150.325, 153.5) -> (-153.5, 150.325) centre (-150.325, 150.325) ccw
  line L649 (-150.325, 153.5) -> (-137.675, 153.5)
  arc A649 (-134.5, 150.325) -> (-137.675, 153.5) centre (-137.675, 150.325) ccw
  line L650 (-134.5, 150.325) -> (-134.5, 137.675)
  arc A650 (-137.675, 134.5) -> (-134.5, 137.675) centre (-137.675, 137.675) ccw
  line L651 (-137.675, 134.5) -> (-150.325, 134.5)
  arc A651 (-153.5, 137.675) -> (-150.325, 134.5) centre (-150.325, 137.675) ccw
  line L652 (-57.5, 137.675) -> (-57.5, 150.325)
  arc A652 (-54.325, 153.5) -> (-57.5, 150.325) centre (-54.325, 150.325) ccw
  line L653 (-54.325, 153.5) -> (-41.675, 153.5)
  arc A653 (-38.5, 150.325) -> (-41.675, 153.5) centre (-41.675, 150.325) ccw
  line L654 (-38.5, 150.325) -> (-38.5, 137.675)
  arc A654 (-41.675, 134.5) -> (-38.5, 137.675) centre (-41.675, 137.675) ccw
  line L655 (-41.675, 134.5) -> (-54.325, 134.5)
  arc A655 (-57.5, 137.675) -> (-54.325, 134.5) centre (-54.325, 137.675) ccw
  line L656 (-129.5, 161.675) -> (-129.5, 174.325)
  arc A656 (-126.325, 177.5) -> (-129.5, 174.325) centre (-126.325, 174.325) ccw
  line L657 (-126.325, 177.5) -> (-113.675, 177.5)
  arc A657 (-110.5, 174.325) -> (-113.675, 177.5) centre (-113.675, 174.325) ccw
  line L658 (-110.5, 174.325) -> (-110.5, 161.675)
  arc A658 (-113.675, 158.5) -> (-110.5, 161.675) centre (-113.675, 161.675) ccw
  line L659 (-113.675, 158.5) -> (-126.325, 158.5)
  arc A659 (-129.5, 161.675) -> (-126.325, 158.5) centre (-126.325, 161.675) ccw
  line L660 (-33.5, 161.675) -> (-33.5, 174.325)
  arc A660 (-30.325, 177.5) -> (-33.5, 174.325) centre (-30.325, 174.325) ccw
  line L661 (-30.325, 177.5) -> (-17.675, 177.5)
  arc A661 (-14.5, 174.325) -> (-17.675, 177.5) centre (-17.675, 174.325) ccw
  line L662 (-14.5, 174.325) -> (-14.5, 161.675)
  arc A662 (-17.675, 158.5) -> (-14.5, 161.675) centre (-17.675, 161.675) ccw
  line L663 (-17.675, 158.5) -> (-30.325, 158.5)
  arc A663 (-33.5, 161.675) -> (-30.325, 158.5) centre (-30.325, 161.675) ccw
  line L664 (110.5, -126.325) -> (110.5, -113.675)
  arc A664 (113.675, -110.5) -> (110.5, -113.675) centre (113.675, -113.675) ccw
  line L665 (113.675, -110.5) -> (126.325, -110.5)
  arc A665 (129.5, -113.675) -> (126.325, -110.5) centre (126.325, -113.675) ccw
  line L666 (129.5, -113.675) -> (129.5, -126.325)
  arc A666 (126.325, -129.5) -> (129.5, -126.325) centre (126.325, -126.325) ccw
  line L667 (126.325, -129.5) -> (113.675, -129.5)
  arc A667 (110.5, -126.325) -> (113.675, -129.5) centre (113.675, -126.325) ccw
  line L668 (110.5, -102.325) -> (110.5, -89.675)
  arc A668 (113.675, -86.5) -> (110.5, -89.675) centre (113.675, -89.675) ccw
  line L669 (113.675, -86.5) -> (126.325, -86.5)
  arc A669 (129.5, -89.675) -> (126.325, -86.5) centre (126.325, -89.675) ccw
  line L670 (129.5, -89.675) -> (129.5, -102.325)
  arc A670 (126.325, -105.5) -> (129.5, -102.325) centre (126.325, -102.325) ccw
  line L671 (126.325, -105.5) -> (113.675, -105.5)
  arc A671 (110.5, -102.325) -> (113.675, -105.5) centre (113.675, -102.325) ccw
  line L672 (-81.5, -102.325) -> (-81.5, -89.675)
  arc A672 (-78.325, -86.5) -> (-81.5, -89.675) centre (-78.325, -89.675) ccw
  line L673 (-78.325, -86.5) -> (-65.675, -86.5)
  arc A673 (-62.5, -89.675) -> (-65.675, -86.5) centre (-65.675, -89.675) ccw
  line L674 (-62.5, -89.675) -> (-62.5, -102.325)
  arc A674 (-65.675, -105.5) -> (-62.5, -102.325) centre (-65.675, -102.325) ccw
  line L675 (-65.675, -105.5) -> (-78.325, -105.5)
  arc A675 (-81.5, -102.325) -> (-78.325, -105.5) centre (-78.325, -102.325) ccw
  line L676 (-57.5, -102.325) -> (-57.5, -89.675)
  arc A676 (-54.325, -86.5) -> (-57.5, -89.675) centre (-54.325, -89.675) ccw
  line L677 (-54.325, -86.5) -> (-41.675, -86.5)
  arc A677 (-38.5, -89.675) -> (-41.675, -86.5) centre (-41.675, -89.675) ccw
  line L678 (-38.5, -89.675) -> (-38.5, -102.325)
  arc A678 (-41.675, -105.5) -> (-38.5, -102.325) centre (-41.675, -102.325) ccw
  line L679 (-41.675, -105.5) -> (-54.325, -105.5)
  arc A679 (-57.5, -102.325) -> (-54.325, -105.5) centre (-54.325, -102.325) ccw
  line L680 (86.5, -102.325) -> (86.5, -89.675)
  arc A680 (89.675, -86.5) -> (86.5, -89.675) centre (89.675, -89.675) ccw
  line L681 (89.675, -86.5) -> (102.325, -86.5)
  arc A681 (105.5, -89.675) -> (102.325, -86.5) centre (102.325, -89.675) ccw
  line L682 (105.5, -89.675) -> (105.5, -102.325)
  arc A682 (102.325, -105.5) -> (105.5, -102.325) centre (102.325, -102.325) ccw
  line L683 (102.325, -105.5) -> (89.675, -105.5)
  arc A683 (86.5, -102.325) -> (89.675, -105.5) centre (89.675, -102.325) ccw
  line L684 (86.5, -126.325) -> (86.5, -113.675)
  arc A684 (89.675, -110.5) -> (86.5, -113.675) centre (89.675, -113.675) ccw
  line L685 (89.675, -110.5) -> (102.325, -110.5)
  arc A685 (105.5, -113.675) -> (102.325, -110.5) centre (102.325, -113.675) ccw
  line L686 (105.5, -113.675) -> (105.5, -126.325)
  arc A686 (102.325, -129.5) -> (105.5, -126.325) centre (102.325, -126.325) ccw
  line L687 (102.325, -129.5) -> (89.675, -129.5)
  arc A687 (86.5, -126.325) -> (89.675, -129.5) centre (89.675, -126.325) ccw
  line L688 (-57.5, 161.675) -> (-57.5, 174.325)
  arc A688 (-54.325, 177.5) -> (-57.5, 174.325) centre (-54.325, 174.325) ccw
  line L689 (-54.325, 177.5) -> (-41.675, 177.5)
  arc A689 (-38.5, 174.325) -> (-41.675, 177.5) centre (-41.675, 174.325) ccw
  line L690 (-38.5, 174.325) -> (-38.5, 161.675)
  arc A690 (-41.675, 158.5) -> (-38.5, 161.675) centre (-41.675, 161.675) ccw
  line L691 (-41.675, 158.5) -> (-54.325, 158.5)
  arc A691 (-57.5, 161.675) -> (-54.325, 158.5) centre (-54.325, 161.675) ccw
  line L692 (-153.5, 161.675) -> (-153.5, 174.325)
  arc A692 (-150.325, 177.5) -> (-153.5, 174.325) centre (-150.325, 174.325) ccw
  line L693 (-150.325, 177.5) -> (-137.675, 177.5)
  arc A693 (-134.5, 174.325) -> (-137.675, 177.5) centre (-137.675, 174.325) ccw
  line L694 (-134.5, 174.325) -> (-134.5, 161.675)
  arc A694 (-137.675, 158.5) -> (-134.5, 161.675) centre (-137.675, 161.675) ccw
  line L695 (-137.675, 158.5) -> (-150.325, 158.5)
  arc A695 (-153.5, 161.675) -> (-150.325, 158.5) centre (-150.325, 161.675) ccw
  line L696 (-81.5, 137.675) -> (-81.5, 150.325)
  arc A696 (-78.325, 153.5) -> (-81.5, 150.325) centre (-78.325, 150.325) ccw
  line L697 (-78.325, 153.5) -> (-65.675, 153.5)
  arc A697 (-62.5, 150.325) -> (-65.675, 153.5) centre (-65.675, 150.325) ccw